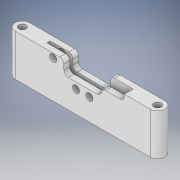
# Autodesk Inventor part: Pixy 2 Halterung
Saved by Autodesk Inventor 2018 (Build 220112000, 112)
## iProperties
Created: 2019-03-05
Part Number: Pixy 2 Halterung
Material: ABS-Kunststoff
Document SubType Name: Modeling
Designer: RedBots
Density: 1.06 g/cm^3
Appearance: Glatt - weiß
Mass: 8.5002 g
Surface Area: 48.1307 cm^2
Volume: 8.01905 cm^3
Author: RedBots
Autodesk Inventor part; units mm, degrees
ref_plane "YZ Plane" through (0, 0, 0) normal (1, 0, 0) x (0, 1, 0)
ref_plane "XZ Plane" through (0, 0, 0) normal (0, 1, 0) x (-1, 0, 0)
sketch "Skizze1" plane through (0, 0, 0) normal (0, 0, 1) x (1, 0, 0)
  circle A0 centre (0, 0) radius 1.75
  circle A1 centre (65, 0) radius 1.75
  line L0 (0, 0) -> (65, 0) construction
  arc A2 (0, 3.5) -> (0, -3.5) centre (0, 0) ccw
  arc A3 (65, -3.5) -> (65, 3.5) centre (65, 0) ccw
  line L1 (0, 3.5) -> (65, 3.5)
  line L2 (65, -3.5) -> (0, -3.5)
  line L3 (0, 3.5) -> (0, -3.5) construction
  line L4 (65, 3.5) -> (65, -3.5) construction
  dimension "d0" = 3.5
  dimension "d1" = 65
  dimension "d2" = 7
  constraints: 10 end point, 5 point on circle, 4 centre point, 4 coincident, 4 tangent, 2 midpoint, 1 equal radius, 1 horizontal, 1 parallel
  measures "d0" diameter of A0
  measures "d1" distance of L0.end L0.start
  measures "d2" distance of L1.end L4.end
extrude "Extrusion1" add sketch "Skizze1" along normal blind 20
ref_plane "Arbeitsebene1" through (0, 0, 0) normal (0, -1, 0) x (1, 0, 0)
ref_plane "Arbeitsebene2" through (65, -3.5, 20) normal (0, -1, 0) x (1, 0, 0)
sketch "Skizze2" plane through (0, 0, 0) normal (0, -1, 0) x (1, 0, 0)
  line L0 (41.5, 13.5) -> (23.5, 13.5) construction
  line L1 (23.5, 13.5) -> (23.5, 7) construction
  line L2 (23.5, 7) -> (41.5, 7)
  line L3 (41.5, 7) -> (41.5, 13.5) construction
  line L4 (21, 13.5) -> (23.5, 11)
  line L5 (23.5, 11) -> (23.5, 13.5) construction
  line L6 (21, 13.5) -> (23.5, 13.5) construction
  line L7 (23.5, 11) -> (23.5, 7)
  line L8 (32.5, 13.5) -> (32.5, 7) construction
  line L9 (44, 13.5) -> (41.5, 11)
  line L10 (44, 13.5) -> (41.5, 13.5) construction
  line L11 (41.5, 11) -> (41.5, 7)
  line L12 (32.5, 13.5) -> (32.5, 20) construction
  line L13 (0, 20) -> (65, 20) construction
  line L14 (21, 13.5) -> (12.5, 13.5)
  line L15 (44, 13.5) -> (52.5, 13.5)
  line L16 (12.5, 13.5) -> (12.5, 20)
  line L17 (52.5, 13.5) -> (52.5, 20)
  line L18 (12.5, 20) -> (52.5, 20)
  point P0 (0, 0)
  dimension "d5" = 18
  dimension "d6" = 6.5
  dimension "d7" = 2.5
  dimension "d11" = 6.5
  dimension "d12" = 40
  constraints: 36 end point, 4 horizontal, 4 vertical, 3 midpoint, 3 perpendicular, 3 point on line, 2 equal length, 2 parallel, 2 symmetric about line
  measures "d5" distance of L2.end L1.end
  measures "d6" distance of L1.end L0.end
  measures "d7" distance of L0.end L4.end
  measures "d11" distance between parallel lines of L13 L0
  measures "d12" distance between parallel lines of L17 L16
extrude "Extrusion2" cut sketch "Skizze2" along normal mid plane 1.5
fillet "Rundung1" radius 1 4 edges at (23.5, 0, 11) (41.5, 0, 11) (21, 0, 13.5) (44, 0, 13.5)
sketch "Skizze3" plane through (0, -3.5, 0) normal (0, -1, 0) x (1, 0, 0)
  line L0 (41.5, 10.5) -> (23.5, 10.5) construction
  circle A0 centre (29.3, 10.5) radius 1.75
  circle A1 centre (35.7, 10.5) radius 1.75
  line L1 (35.7, 10.5) -> (29.3, 10.5) construction
  line L2 (29.3, 10.5) -> (29.3, 18) construction
  line L3 (29.3, 18) -> (18.325, 18) construction
  circle A2 centre (18.325, 18) radius 1.75
  line L4 (23.5, 10.5858) -> (23.5, 7) projected
  line L5 (41.5, 7) -> (41.5, 10.5858) projected
  line L6 (23.5, 7) -> (41.5, 7) projected
  point P0 (0, 0)
  point P1 (32.5, 10.5)
  dimension "d13" = 3.5
  dimension "d14" = 6.4
  dimension "d22" = 7.5
  dimension "d23" = 10.975
  dimension "d25" = 3.5
  constraints: 8 end point, 4 point on line, 3 centre point, 2 equal radius, 2 midpoint, 2 perpendicular, 1 coincident, 1 horizontal
  measures "d13" diameter of A0
  measures "d14" distance of L1.start L1.end
  measures "d22" distance of L1.end L2.end
  measures "d23" distance of L2.end L3.end
  measures "d25" distance between parallel lines of L6 L0
extrude "Extrusion3" cut sketch "Skizze3" against normal through all
sketch "Skizze5" plane through (0, 0, 20) normal (0, 0, 1) x (1, 0, 0)
  line L0 (65, 3.5) -> (0, 3.5) projected
  line L1 (41.5, 3.5) -> (23.5, 3.5)
  line L2 (23.5, 3.5) -> (23.5, 0.75)
  line L3 (23.5, 0.75) -> (41.5, 0.75)
  line L4 (41.5, 0.75) -> (41.5, 3.5)
  point P0 (0, 0)
  point P1 (32.5, 3.5)
  constraints: 8 end point, 2 midpoint, 2 parallel, 1 coincident, 1 horizontal, 1 perpendicular, 1 point on line
extrude "Extrusion5" cut sketch "Skizze5" against normal up to surface (6.5 mm away)
sketch "Skizze6" plane through (0, -3.5, 0) normal (0, -1, 0) x (1, 0, 0)
  line L0 (52.5, 13.5) -> (52.5, 20) projected
  line L1 (52.5, 20) -> (41.5, 20)
  line L2 (41.5, 20) -> (41.5, 17)
  line L3 (41.5, 17) -> (52.5, 17)
  line L4 (52.5, 17) -> (52.5, 20)
  line L5 (23.5, 13.5) -> (23.5, 20) projected
  line L6 (41.5, 20) -> (23.5, 20)
  line L7 (23.5, 20) -> (23.5, 13.5)
  line L8 (23.5, 13.5) -> (41.5, 13.5)
  line L9 (41.5, 13.5) -> (41.5, 20)
  point P0 (0, 0)
  dimension "d26" = 3
  constraints: 16 end point, 4 parallel, 2 horizontal, 2 perpendicular, 2 point on line
  measures "d26" distance of L1.end L2.end
extrude "Extrusion6" cut sketch "Skizze6" against normal up to surface (2.75 mm away)
fillet "Rundung2" radius 2 9 edges at (41.5, -2.125, 17) (52.5, -2.125, 17) (41.5, -2.125, 13.5) (23.5, -2.125, 13.5) (23.5, -2.125, 20) (23.5, 2.125, 13.5) (23.5, 2.125, 20) (41.5, 2.125, 13.5) (41.5, 2.125, 20)
